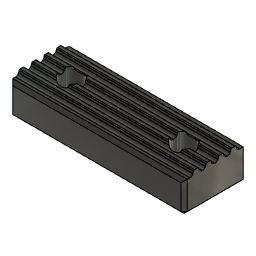
Belt_Fixture (Autodesk Fusion 360 design; units mm, degrees)
Autodesk Fusion 360 part; units mm, degrees
note: some values were not read from the file. Chosen so that the rebuilt part matches the saved one: which face or edge a step refers to. Set by a fixed rule: which sketch regions a step uses.
sketch "Sketch3" plane through (0, 0, -8) normal (0, 0, -1) x (1, 0, 0)
  line L0 (-18.54, -15) -> (0.5, -15)
  line L1 (0.5, -15) -> (-18.54, -15)
  line L2 (0.5, -24.0722) -> (-17.5611, -24.0722)
  line L3 (-17.5611, -24.0722) -> (0.5, -24.0722)
  circle A0 centre (0, -19) radius 1.75
  circle A1 centre (0, -19) radius 1.75
  circle A2 centre (-18.04, -19) radius 1.75
  circle A3 centre (-18.04, -19) radius 1.75
  line L4 (-23.0745, -14.0722) -> (4.9255, -14.0722)
  line L5 (4.9255, -14.0722) -> (4.9255, -24.0722)
  line L6 (4.9255, -24.0722) -> (-23.0745, -24.0722)
  line L7 (-23.0745, -24.0722) -> (-23.0745, -14.0722)
  dimension "d1" = 28
  dimension "d2" = 10
  constraint horizontal L4
  constraint vertical L5
  constraint horizontal L6
  constraint vertical L7
  constraint coincident L2.start L6
  measures "d1" distance of L5 L7
  measures "d2" distance of L3 L4
extrude "Extrude1" add sketch "Sketch3" along normal blind 5
move_face "MoveFace1" by (0, 5, 0) 1 faces at (-23.0745, 20.7388, -9.6667)
sketch "Sketch2" plane through (3, 0, 0) normal (1, 0, 0) x (0, 1, 0)
  circle A0 centre (17, -7.445) radius 0.555
  line L0 (-21.5067, -8) -> (16, -8) construction
  line L1 (-21.5067, -6.62) -> (16, -6.62) construction
  line L2 (16, -8) -> (16, -6.62) construction
  line L3 (-21.5067, -7.25) -> (16, -7.25) construction
  line L4 (-21.5067, -6.62) -> (-21.5067, -8) construction
  line L5 (-21.5067, -6.996) -> (16, -6.996) construction
  line L6 (17, -8) -> (17, -6.62) construction
  circle A1 centre (17.4, -7.25) radius 1
  circle A2 centre (14.6, -7.25) radius 1 construction
  circle A3 centre (15, -7.445) radius 0.555 construction
  line L7 (15, -7.445) -> (17, -7.445) construction
  circle A4 centre (16.2598, -7.4) radius 0.15
  circle A5 centre (15.7402, -7.4) radius 0.15
  circle A6 centre (15, -7.445) radius 0.555
  circle A7 centre (14.6, -7.25) radius 1
  line L8 (15.7402, -7.25) -> (16.2598, -7.25)
  line L9 (15, -8) -> (17, -8)
  line L10 (20.5, -8) -> (17.5, -8)
  line L11 (17.5, -8) -> (17.5, -13)
  line L12 (17.5, -13) -> (20.5, -13)
  line L13 (20.5, -13) -> (20.5, -8)
  point P0 (17.4, -7.25)
  point P1 (15, -8)
  dimension "d356" = 1.11
  dimension "d357" = 1.38
  dimension "d358" = 0.75
  dimension "d359" = 0.254
  dimension "d360" = 0.4
  dimension "d361" = 2
  dimension "d362" = 1
  dimension "d363" = 0.3
  constraint horizontal L0
  constraint tangent A0 L0
  constraint horizontal L1
  constraint vertical L2
  constraint coincident L2 L3.end
  constraint perpendicular L2 L3
  constraint vertical L4
  constraint coincident L3.start L4
  constraint coincident L0.start L4.end
  constraint coincident L4 L5.start
  constraint coincident L2 L5.end
  constraint perpendicular L2 L5
  constraint perpendicular L1 L6
  constraint coincident A0 L6.start
  constraint coincident L0 L6.start
  constraint coincident L1 L6.end
  constraint coincident L3 P0
  constraint coincident P0 A1.centre
  constraint symmetric A0 L2 A3
  constraint symmetric L2 A1 A2
  constraint coincident A3.centre L7.start
  constraint coincident A0.centre L7.end
  constraint tangent L3 A4
  constraint tangent A1 A4
  constraint symmetric A0 L2 A6
  constraint symmetric L2 A1 A7
  constraint symmetric L2 A4 A5
  constraint coincident A5 L8.start
  constraint coincident A4 L8.end
  constraint tangent A5 L8
  constraint tangent A4 L8
  constraint coincident A3 P1
  constraint tangent A3 L9
  constraint tangent A0 L9
  constraint coincident L9 P1
  measures "d356" diameter of A0
  measures "d357" distance of L0 L1
  measures "d358" distance of L0 L3
  measures "d359" distance of L3 L5
  measures "d360" distance of L6 P0
  measures "d361" diameter of A1
  measures "d362" distance of L2 L6
  measures "d363" diameter of A4
extrude "Extrude2" add sketch "Sketch2" along normal up to surface (1.9255 mm away) and the other way up to surface (26.0745 mm away) contours A0 A1 L9 | A4 | A1 A4 A5 A7 L8 L9 | A6 A7 L9 | A5 picked at (15.2605, -7.9559)
sketch "Sketch5" plane through (-23.0745, 0, 0) normal (-1, 0, 0) x (0, -1, 0)
  line L0 (-17, -8) -> (-24.0722, -8)
  line L1 (-24.0722, -8) -> (-24.0722, -13)
  line L2 (-24.0722, -13) -> (-14.0722, -13)
  line L3 (-14.0722, -13) -> (-14.0722, -8)
  line L4 (-14.0722, -8) -> (-15, -8)
  arc A0 (-15.4995, -7.6869) -> (-15, -8) centre (-15, -7.445) ccw
  arc A1 (-15.5915, -7.3804) -> (-15.4995, -7.6869) centre (-14.6, -7.25) ccw
  arc A2 (-15.5915, -7.3804) -> (-15.7402, -7.25) centre (-15.7402, -7.4) ccw
  line L5 (-15.7402, -7.25) -> (-16.2598, -7.25)
  arc A3 (-16.2598, -7.25) -> (-16.4085, -7.3804) centre (-16.2598, -7.4) ccw
  arc A4 (-16.5005, -7.6869) -> (-16.4085, -7.3804) centre (-17.4, -7.25) ccw
  arc A5 (-17, -8) -> (-16.5005, -7.6869) centre (-17, -7.445) ccw
pattern_linear "R-Pattern1" count 4 spacing 2 along (0, 1, 0) of "Extrude2"
extrude "Extrude3" cut sketch "Sketch3" against normal blind 5 contours A0 A1 | A2 A3
extrude "Extrude4" cut sketch "Sketch3" against normal blind 5 contours A0 A1 | A2 A3
sketch "Sketch4" plane through (0, 0, -13) normal (0, 0, -1) x (1, 0, 0)
  line L0 (-15.24, -17.3834) -> (-18.04, -15.7668)
  line L1 (-18.04, -15.7668) -> (-20.84, -17.3834)
  line L2 (-20.84, -17.3834) -> (-20.84, -20.6166)
  line L3 (-20.84, -20.6166) -> (-18.04, -22.2332)
  line L4 (-18.04, -22.2332) -> (-15.24, -20.6166)
  line L5 (-15.24, -20.6166) -> (-15.24, -17.3834)
  line L6 (-2.8, -20.6166) -> (0, -22.2332)
  line L7 (0, -22.2332) -> (2.8, -20.6166)
  line L8 (2.8, -20.6166) -> (2.8, -17.3834)
  line L9 (2.8, -17.3834) -> (0, -15.7668)
  line L10 (0, -15.7668) -> (-2.8, -17.3834)
  line L11 (-2.8, -17.3834) -> (-2.8, -20.6166)
  circle A0 centre (-18.04, -19) radius 1.75
  circle A1 centre (0, -19) radius 1.75
  line L12 (-23.0745, -24.0722) -> (4.9255, -24.0722)
  line L13 (-23.0745, -24.0722) -> (-23.0745, -14.0722)
  line L14 (4.9255, -24.0722) -> (4.9255, -14.0722)
  line L15 (-23.0745, -14.0722) -> (-23.0745, -24.0722)
  line L16 (4.9255, -14.0722) -> (-23.0745, -14.0722)
  point P0 (-18.04, -19)
  point P1 (0, -19)
  dimension "d462" = 2.8
  dimension "d463" = 2.8
  constraint parallel L5 L11
  constraint parallel L2 L13
  constraint coincident P0 A0.centre
  constraint coincident P1 A1.centre
  measures "d462" distance of P0 L5
  measures "d463" distance of P1 L11
extrude "Extrude5" cut sketch "Sketch4" against normal blind 2.5 contours L0 L1 L2 L3 L4 L5 | L6 L7 L8 L9 L10 L11
chamfer "Chamfer3" distance 0.5 angle 45 2 edges at (4.9255, 19.0722, -13) (-9.0745, 24.0722, -13)
chamfer "Chamfer3" distance 0.5 angle 45 1 edges at (-23.0745, 14.0722, -10.5)
chamfer "Chamfer3" distance 0.5 angle 45 1 edges at (-23.0745, 24.0722, -10.5)
chamfer "Chamfer3" distance 0.5 angle 45 4 edges at (4.9255, 14.0722, -10.5) (4.9255, 24.0722, -10.5) (-9.0745, 24.0722, -8) (-9.0745, 14.0722, -8)
chamfer "Chamfer3" distance 0.5 angle 45 1 edges at (-9.0745, 14.0722, -13)
chamfer "Chamfer3" distance 0.5 angle 45 1 edges at (-23.0745, 19.0722, -13)
equation "d356 = GT_R3 * 2"
equation "d357 = GT_H"
equation "d358 = GT_h"
equation "d359 = GT_PLD"
equation "d360 = GT_b"
equation "d361 = GT_R2 * 2"
equation "d362 = GT_P / 2"
equation "d363 = GT_R1 * 2"
equation "GT_H = 1.38 mm"
equation "GT_R1 = 0.15 mm"
equation "GT_R2 = 1 mm"
equation "GT_R3 = 0.555 mm"
equation "GT_h = 0.75 mm"
equation "GT_P = 2 mm"
equation "GT_b = 0.40 mm"
equation "GT_PLD = 0.254 mm"
